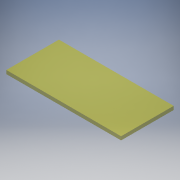
# Autodesk Inventor part: frontBox
Saved by Autodesk Inventor 2016 SP1 (Build 200210100, 210)
## iProperties
Created: 2016-01-20
Part Number: frontBox
Material: Generic
Document SubType Name: Modeling
Designer: steele
Density: 1 g/cm^3
Appearance: Clear - Yellow
Author: steele
Autodesk Inventor part; units mm, degrees
ref_plane "YZ Plane" through (0, 0, 0) normal (1, 0, 0) x (0, 1, 0)
ref_plane "XZ Plane" through (0, 0, 0) normal (0, 1, 0) x (-1, 0, 0)
ref_plane "XY Plane" through (0, 0, 0) normal (0, 0, 1) x (1, 0, 0)
sketch "Sketch1" plane through (0, 0, 0) normal (0, 1, 0) x (-1, 0, 0)
  line L0 (304.8, 139.7) -> (-304.8, 139.7)
  line L1 (-304.8, 139.7) -> (-304.8, -139.7)
  line L2 (-304.8, -139.7) -> (304.8, -139.7)
  line L3 (304.8, -139.7) -> (304.8, 139.7)
  line L4 (304.8, 139.7) -> (-304.8, -139.7) construction
  line L5 (-304.8, 139.7) -> (304.8, -139.7) construction
  point P0 (0, 0)
  dimension "d0" = 609.6
  dimension "d1" = 279.4
  constraints: 12 end point, 2 midpoint, 2 parallel, 1 horizontal, 1 perpendicular
  measures "d0" distance of L0.start L0.end
  measures "d1" distance of L0.end L1.end
extrude "Extrusion1" add sketch "Sketch1" along normal blind 19.05
equation "\"d0\" = frontBoxWidth"
equation "\"d1\" = frontBoxLength"
equation "\"d2\" = frontBoxThickness"
equation "\"frontBoxWidth\" = 609.6"
equation "\"frontBoxLength\" = 279.4"
equation "\"frontBoxThickness\" = 19.05"
body "Solid1"
